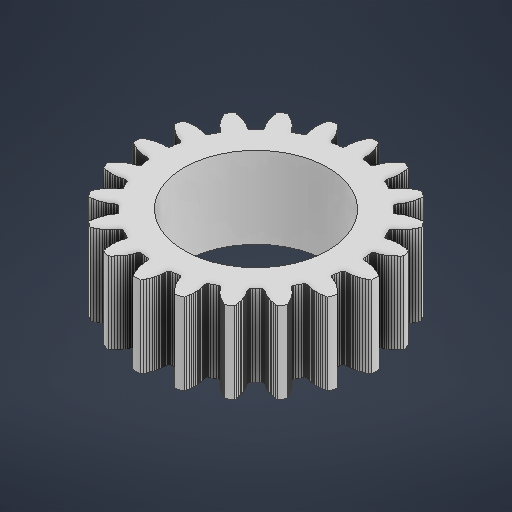
# Autodesk Inventor part: pole_gear_v2
Saved by Autodesk Inventor 2026.2 (Build 302298000, 298)
## iProperties
Created: 2026-01-14
Part Number: pole_gear_v2
Material: Generic
Document SubType Name: Modeling
Designer: User
Density: 1 g/cm^3
Appearance: Default
Author: User
Autodesk Inventor part; units mm, degrees
(part 1 of 3)
ref_plane "YZ Plane" through (0, 0, 0) normal (1, 0, 0) x (0, 1, 0)
ref_plane "XZ Plane" through (0, 0, 0) normal (0, 1, 0) x (-1, 0, 0)
ref_plane "XY Plane" through (0, 0, 0) normal (0, 0, 1) x (1, 0, 0)
sketch "Sketch1" plane through (0, 0, 0) normal (0, 1, 0) x (-1, 0, 0)
  circle A0 centre (0, 0) radius 13.25
  circle A1 centre (0, 0) radius 13.25
  line L0 (20.839, 5.8308) -> (20.5291, 5.5298)
  line L1 (20.5291, 5.5298) -> (20.2304, 5.263)
  line L2 (20.2304, 5.263) -> (19.9477, 5.0311)
  line L3 (19.9477, 5.0311) -> (19.6809, 4.8302)
  line L4 (19.6809, 4.8302) -> (19.4329, 4.6593)
  line L5 (19.4329, 4.6593) -> (19.2065, 4.5169)
  line L6 (19.2065, 4.5169) -> (19.0014, 4.3995)
  line L7 (19.0014, 4.3995) -> (18.8229, 4.307)
  line L8 (18.8229, 4.307) -> (18.5448, 4.1835)
  line L9 (18.5448, 4.1835) -> (18.3792, 4.1257)
  line L10 (18.3792, 4.1257) -> (18.2149, 4.0764)
  line L11 (18.2149, 4.0764) -> (18.015, 3.9979)
  line L12 (18.015, 3.9979) -> (17.8537, 3.9113)
  line L13 (17.8537, 3.9113) -> (17.7876, 3.866)
  line L14 (17.7876, 3.866) -> (17.7313, 3.8197)
  line L15 (17.7313, 3.8197) -> (17.6846, 3.773)
  line L16 (17.6846, 3.773) -> (17.6477, 3.7262)
  line L17 (17.6477, 3.7262) -> (17.6205, 3.6797)
  line L18 (17.6205, 3.6797) -> (17.6029, 3.6338)
  line L19 (17.6029, 3.6338) -> (17.5949, 3.589)
  line L20 (17.5949, 3.589) -> (17.5985, 3.5351)
  line L21 (17.5985, 3.5351) -> (17.6581, 3.2242)
  line L22 (17.6581, 3.2242) -> (17.729, 2.808)
  line L23 (17.729, 2.808) -> (17.7902, 2.3902)
  line L24 (17.7902, 2.3902) -> (17.8295, 2.0761)
  line L25 (17.8295, 2.0761) -> (17.8429, 2.0238)
  line L26 (17.8429, 2.0238) -> (17.8643, 1.9836)
  line L27 (17.8643, 1.9836) -> (17.8951, 1.9454)
  line L28 (17.8951, 1.9454) -> (17.9354, 1.9096)
  line L29 (17.9354, 1.9096) -> (17.985, 1.8765)
  line L30 (17.985, 1.8765) -> (18.0438, 1.8465)
  line L31 (18.0438, 1.8465) -> (18.1117, 1.8199)
  line L32 (18.1117, 1.8199) -> (18.1886, 1.7972)
  line L33 (18.1886, 1.7972) -> (18.3687, 1.7647)
  line L34 (18.3687, 1.7647) -> (18.583, 1.7518)
  line L35 (18.583, 1.7518) -> (18.7546, 1.7557)
  line L36 (18.7546, 1.7557) -> (18.9299, 1.7519)
  line L37 (18.9299, 1.7519) -> (19.2325, 1.7204)
  line L38 (19.2325, 1.7204) -> (19.4309, 1.6876)
  line L39 (19.4309, 1.6876) -> (19.6623, 1.6393)
  line L40 (19.6623, 1.6393) -> (19.9216, 1.5738)
  line L41 (19.9216, 1.5738) -> (20.2103, 1.4879)
  line L42 (20.2103, 1.4879) -> (20.5261, 1.3793)
  line L43 (20.5261, 1.3793) -> (20.8666, 1.2461)
  line L44 (20.8666, 1.2461) -> (21.2331, 1.0847)
  line L45 (21.2331, 1.0847) -> (21.6209, 0.8942)
  line L46 (21.6209, 0.8942) -> (21.989, 0.6945)
  arc A2 (21.989, -0.6945) -> (21.989, 0.6945) centre (0, 0) ccw
  line L47 (21.989, -0.6945) -> (21.6209, -0.8942)
  line L48 (21.6209, -0.8942) -> (21.2331, -1.0847)
  line L49 (21.2331, -1.0847) -> (20.8666, -1.2461)
  line L50 (20.8666, -1.2461) -> (20.5261, -1.3793)
  line L51 (20.5261, -1.3793) -> (20.2103, -1.4879)
  line L52 (20.2103, -1.4879) -> (19.9216, -1.5738)
  line L53 (19.9216, -1.5738) -> (19.6623, -1.6393)
  line L54 (19.6623, -1.6393) -> (19.4309, -1.6876)
  line L55 (19.4309, -1.6876) -> (19.2325, -1.7204)
  line L56 (19.2325, -1.7204) -> (18.9299, -1.7519)
  line L57 (18.9299, -1.7519) -> (18.7546, -1.7557)
  line L58 (18.7546, -1.7557) -> (18.583, -1.7518)
  line L59 (18.583, -1.7518) -> (18.3687, -1.7647)
  line L60 (18.3687, -1.7647) -> (18.1886, -1.7972)
  line L61 (18.1886, -1.7972) -> (18.1117, -1.8199)
  line L62 (18.1117, -1.8199) -> (18.0438, -1.8465)
  line L63 (18.0438, -1.8465) -> (17.985, -1.8765)
  line L64 (17.985, -1.8765) -> (17.9354, -1.9096)
  line L65 (17.9354, -1.9096) -> (17.8951, -1.9454)
  line L66 (17.8951, -1.9454) -> (17.8643, -1.9836)
  line L67 (17.8643, -1.9836) -> (17.8429, -2.0238)
  line L68 (17.8429, -2.0238) -> (17.8295, -2.0761)
  line L69 (17.8295, -2.0761) -> (17.7902, -2.3902)
  line L70 (17.7902, -2.3902) -> (17.729, -2.808)
  line L71 (17.729, -2.808) -> (17.6581, -3.2242)
  line L72 (17.6581, -3.2242) -> (17.5985, -3.5351)
  line L73 (17.5985, -3.5351) -> (17.5949, -3.589)
  line L74 (17.5949, -3.589) -> (17.6029, -3.6338)
  line L75 (17.6029, -3.6338) -> (17.6205, -3.6797)
  line L76 (17.6205, -3.6797) -> (17.6477, -3.7262)
  line L77 (17.6477, -3.7262) -> (17.6846, -3.773)
  line L78 (17.6846, -3.773) -> (17.7313, -3.8197)
  line L79 (17.7313, -3.8197) -> (17.7876, -3.866)
  line L80 (17.7876, -3.866) -> (17.8537, -3.9113)
  line L81 (17.8537, -3.9113) -> (18.015, -3.9979)
  line L82 (18.015, -3.9979) -> (18.2149, -4.0764)
  line L83 (18.2149, -4.0764) -> (18.3792, -4.1257)
  line L84 (18.3792, -4.1257) -> (18.5448, -4.1835)
  line L85 (18.5448, -4.1835) -> (18.8229, -4.307)
  line L86 (18.8229, -4.307) -> (19.0014, -4.3995)
  line L87 (19.0014, -4.3995) -> (19.2065, -4.5169)
  line L88 (19.2065, -4.5169) -> (19.4329, -4.6593)
  line L89 (19.4329, -4.6593) -> (19.6809, -4.8302)
  line L90 (19.6809, -4.8302) -> (19.9477, -5.0311)
  line L91 (19.9477, -5.0311) -> (20.2304, -5.263)
  line L92 (20.2304, -5.263) -> (20.5291, -5.5298)
  line L93 (20.5291, -5.5298) -> (20.839, -5.8308)
  line L94 (20.839, -5.8308) -> (21.1274, -6.1345)
  arc A3 (20.6982, -7.4555) -> (21.1274, -6.1345) centre (0, 0) ccw
  line L95 (20.6982, -7.4555) -> (20.2864, -7.5317)
  line L96 (20.2864, -7.5317) -> (19.8587, -7.593)
  line L97 (19.8587, -7.593) -> (19.4602, -7.6332)
  line L98 (19.4602, -7.6332) -> (19.0953, -7.6547)
  line L99 (19.0953, -7.6547) -> (18.7613, -7.6604)
  line L100 (18.7613, -7.6604) -> (18.4602, -7.6529)
  line L101 (18.4602, -7.6529) -> (18.1934, -7.6351)
  line L102 (18.1934, -7.6351) -> (17.9584, -7.6095)
  line L103 (17.9584, -7.6095) -> (17.7596, -7.5794)
  line L104 (17.7596, -7.5794) -> (17.462, -7.5158)
  line L105 (17.462, -7.5158) -> (17.2942, -7.4653)
  line L106 (17.2942, -7.4653) -> (17.1322, -7.4085)
  line L107 (17.1322, -7.4085) -> (16.9244, -7.3546)
  line L108 (16.9244, -7.3546) -> (16.743, -7.3298)
  line L109 (16.743, -7.3298) -> (16.6629, -7.3277)
  line L110 (16.6629, -7.3277) -> (16.5901, -7.3319)
  line L111 (16.5901, -7.3319) -> (16.5249, -7.3423)
  line L112 (16.5249, -7.3423) -> (16.4675, -7.3585)
  line L113 (16.4675, -7.3585) -> (16.4181, -7.3801)
  line L114 (16.4181, -7.3801) -> (16.3769, -7.4069)
  line L115 (16.3769, -7.4069) -> (16.3442, -7.4385)
  line L116 (16.3442, -7.4385) -> (16.3153, -7.4841)
  line L117 (16.3153, -7.4841) -> (16.1809, -7.7707)
  line L118 (16.1809, -7.7707) -> (15.9936, -8.1491)
  line L119 (15.9936, -8.1491) -> (15.7975, -8.5231)
  line L120 (15.7975, -8.5231) -> (15.6447, -8.8003)
  line L121 (15.6447, -8.8003) -> (15.6247, -8.8505)
  line L122 (15.6247, -8.8505) -> (15.6184, -8.8956)
  line L123 (15.6184, -8.8956) -> (15.621, -8.9446)
  line L124 (15.621, -8.9446) -> (15.6325, -8.9973)
  line L125 (15.6325, -8.9973) -> (15.6531, -9.0532)
  line L126 (15.6531, -9.0532) -> (15.6831, -9.112)
  line L127 (15.6831, -9.112) -> (15.7224, -9.1734)
  line L128 (15.7224, -9.1734) -> (15.7712, -9.237)
  line L129 (15.7712, -9.237) -> (15.8979, -9.3692)
  line L130 (15.8979, -9.3692) -> (16.0637, -9.5056)
  line L131 (16.0637, -9.5056) -> (16.2048, -9.6033)
  line L132 (16.2048, -9.6033) -> (16.3443, -9.7094)
  line L133 (16.3443, -9.7094) -> (16.5707, -9.9128)
  line L134 (16.5707, -9.9128) -> (16.7119, -10.0559)
  line L135 (16.7119, -10.0559) -> (16.8707, -10.231)
  line L136 (16.8707, -10.231) -> (17.042, -10.4364)
  line L137 (17.042, -10.4364) -> (17.225, -10.6756)
  line L138 (17.225, -10.6756) -> (17.4167, -10.9491)
  line L139 (17.4167, -10.9491) -> (17.6139, -11.257)
  line L140 (17.6139, -11.257) -> (17.8155, -11.603)
  line L141 (17.8155, -11.603) -> (18.0173, -11.985)
  line L142 (18.0173, -11.985) -> (18.1977, -12.3629)
  arc A4 (17.3813, -13.4867) -> (18.1977, -12.3629) centre (0, 0) ccw
  line L143 (17.3813, -13.4867) -> (16.9661, -13.4319)
  line L144 (16.9661, -13.4319) -> (16.5404, -13.3581)
  line L145 (16.5404, -13.3581) -> (16.149, -13.2732)
  line L146 (16.149, -13.2732) -> (15.7953, -13.1808)
  line L147 (15.7953, -13.1808) -> (15.4759, -13.083)
  line L148 (15.4759, -13.083) -> (15.1918, -12.9829)
  line L149 (15.1918, -12.9829) -> (14.9436, -12.8835)
  line L150 (14.9436, -12.8835) -> (14.728, -12.7865)
  line L151 (14.728, -12.7865) -> (14.5482, -12.6964)
  line L152 (14.5482, -12.6964) -> (14.2849, -12.544)
  line L153 (14.2849, -12.544) -> (14.1408, -12.4441)
  line L154 (14.1408, -12.4441) -> (14.0043, -12.3401)
  line L155 (14.0043, -12.3401) -> (13.8234, -12.2245)
  line L156 (13.8234, -12.2245) -> (13.6585, -12.1449)
  line L157 (13.6585, -12.1449) -> (13.5829, -12.1181)
  line L158 (13.5829, -12.1181) -> (13.5124, -12.0997)
  line L159 (13.5124, -12.0997) -> (13.4472, -12.0894)
  line L160 (13.4472, -12.0894) -> (13.3876, -12.0871)
  line L161 (13.3876, -12.0871) -> (13.334, -12.0924)
  line L162 (13.334, -12.0924) -> (13.2865, -12.1051)
  line L163 (13.2865, -12.1051) -> (13.2456, -12.125)
  line L164 (13.2456, -12.125) -> (13.2041, -12.1596)
  line L165 (13.2041, -12.1596) -> (12.9876, -12.3906)
  line L166 (12.9876, -12.3906) -> (12.6926, -12.6926)
  line L167 (12.6926, -12.6926) -> (12.3906, -12.9876)
  line L168 (12.3906, -12.9876) -> (12.1596, -13.2041)
  line L169 (12.1596, -13.2041) -> (12.125, -13.2456)
  line L170 (12.125, -13.2456) -> (12.1051, -13.2865)
  line L171 (12.1051, -13.2865) -> (12.0924, -13.334)
  line L172 (12.0924, -13.334) -> (12.0871, -13.3876)
  line L173 (12.0871, -13.3876) -> (12.0894, -13.4472)
  line L174 (12.0894, -13.4472) -> (12.0997, -13.5124)
  line L175 (12.0997, -13.5124) -> (12.1181, -13.5829)
  line L176 (12.1181, -13.5829) -> (12.1449, -13.6585)
  line L177 (12.1449, -13.6585) -> (12.2245, -13.8234)
  line L178 (12.2245, -13.8234) -> (12.3401, -14.0043)
  line L179 (12.3401, -14.0043) -> (12.4441, -14.1408)
  line L180 (12.4441, -14.1408) -> (12.544, -14.2849)
  line L181 (12.544, -14.2849) -> (12.6964, -14.5482)
  line L182 (12.6964, -14.5482) -> (12.7865, -14.728)
  line L183 (12.7865, -14.728) -> (12.8835, -14.9436)
  line L184 (12.8835, -14.9436) -> (12.9829, -15.1918)
  line L185 (12.9829, -15.1918) -> (13.083, -15.4759)
  line L186 (13.083, -15.4759) -> (13.1808, -15.7953)
  line L187 (13.1808, -15.7953) -> (13.2732, -16.149)
  line L188 (13.2732, -16.149) -> (13.3581, -16.5404)
  line L189 (13.3581, -16.5404) -> (13.4319, -16.9661)
  line L190 (13.4319, -16.9661) -> (13.4867, -17.3813)
  arc A5 (12.3629, -18.1977) -> (13.4867, -17.3813) centre (0, 0) ccw
  line L191 (12.3629, -18.1977) -> (11.985, -18.0173)
  line L192 (11.985, -18.0173) -> (11.603, -17.8155)
  line L193 (11.603, -17.8155) -> (11.257, -17.6139)
  line L194 (11.257, -17.6139) -> (10.9491, -17.4167)
  line L195 (10.9491, -17.4167) -> (10.6756, -17.225)
  line L196 (10.6756, -17.225) -> (10.4364, -17.042)
  line L197 (10.4364, -17.042) -> (10.231, -16.8707)
  line L198 (10.231, -16.8707) -> (10.0559, -16.7119)
  line L199 (10.0559, -16.7119) -> (9.9128, -16.5707)
  line L200 (9.9128, -16.5707) -> (9.7094, -16.3443)
  line L201 (9.7094, -16.3443) -> (9.6033, -16.2048)
  line L202 (9.6033, -16.2048) -> (9.5056, -16.0637)
  line L203 (9.5056, -16.0637) -> (9.3692, -15.8979)
  line L204 (9.3692, -15.8979) -> (9.237, -15.7712)
  line L205 (9.237, -15.7712) -> (9.1734, -15.7224)
  line L206 (9.1734, -15.7224) -> (9.112, -15.6831)
  line L207 (9.112, -15.6831) -> (9.0532, -15.6531)
  line L208 (9.0532, -15.6531) -> (8.9973, -15.6325)
  line L209 (8.9973, -15.6325) -> (8.9446, -15.621)
  line L210 (8.9446, -15.621) -> (8.8956, -15.6184)
  line L211 (8.8956, -15.6184) -> (8.8505, -15.6247)
  line L212 (8.8505, -15.6247) -> (8.8003, -15.6447)
  line L213 (8.8003, -15.6447) -> (8.5231, -15.7975)
  line L214 (8.5231, -15.7975) -> (8.1491, -15.9936)
  line L215 (8.1491, -15.9936) -> (7.7707, -16.1809)
  line L216 (7.7707, -16.1809) -> (7.4841, -16.3153)
  line L217 (7.4841, -16.3153) -> (7.4385, -16.3442)
  line L218 (7.4385, -16.3442) -> (7.4069, -16.3769)
  line L219 (7.4069, -16.3769) -> (7.3801, -16.4181)
  line L220 (7.3801, -16.4181) -> (7.3585, -16.4675)
  line L221 (7.3585, -16.4675) -> (7.3423, -16.5249)
  line L222 (7.3423, -16.5249) -> (7.3319, -16.5901)
  line L223 (7.3319, -16.5901) -> (7.3277, -16.6629)
  line L224 (7.3277, -16.6629) -> (7.3298, -16.743)
  line L225 (7.3298, -16.743) -> (7.3546, -16.9244)
  line L226 (7.3546, -16.9244) -> (7.4085, -17.1322)
  line L227 (7.4085, -17.1322) -> (7.4653, -17.2942)
  line L228 (7.4653, -17.2942) -> (7.5158, -17.462)
  line L229 (7.5158, -17.462) -> (7.5794, -17.7596)
  line L230 (7.5794, -17.7596) -> (7.6095, -17.9584)
  line L231 (7.6095, -17.9584) -> (7.6351, -18.1934)
  line L232 (7.6351, -18.1934) -> (7.6529, -18.4602)
  line L233 (7.6529, -18.4602) -> (7.6604, -18.7613)
  line L234 (7.6604, -18.7613) -> (7.6547, -19.0953)
  line L235 (7.6547, -19.0953) -> (7.6332, -19.4602)
  line L236 (7.6332, -19.4602) -> (7.593, -19.8587)
  line L237 (7.593, -19.8587) -> (7.5317, -20.2864)
  line L238 (7.5317, -20.2864) -> (7.4555, -20.6982)
  arc A6 (6.1345, -21.1274) -> (7.4555, -20.6982) centre (0, 0) ccw
  line L239 (6.1345, -21.1274) -> (5.8308, -20.839)
  line L240 (5.8308, -20.839) -> (5.5298, -20.5291)
  line L241 (5.5298, -20.5291) -> (5.263, -20.2304)
  line L242 (5.263, -20.2304) -> (5.0311, -19.9477)
  line L243 (5.0311, -19.9477) -> (4.8302, -19.6809)
  line L244 (4.8302, -19.6809) -> (4.6593, -19.4329)
  line L245 (4.6593, -19.4329) -> (4.5169, -19.2065)
  line L246 (4.5169, -19.2065) -> (4.3995, -19.0014)
  line L247 (4.3995, -19.0014) -> (4.307, -18.8229)
  line L248 (4.307, -18.8229) -> (4.1835, -18.5448)
  line L249 (4.1835, -18.5448) -> (4.1257, -18.3792)
  line L250 (4.1257, -18.3792) -> (4.0764, -18.2149)
  line L251 (4.0764, -18.2149) -> (3.9979, -18.015)
  line L252 (3.9979, -18.015) -> (3.9113, -17.8537)
  line L253 (3.9113, -17.8537) -> (3.866, -17.7876)
  line L254 (3.866, -17.7876) -> (3.8197, -17.7313)
  line L255 (3.8197, -17.7313) -> (3.773, -17.6846)
  line L256 (3.773, -17.6846) -> (3.7262, -17.6477)
  line L257 (3.7262, -17.6477) -> (3.6797, -17.6205)
  line L258 (3.6797, -17.6205) -> (3.6338, -17.6029)
  line L259 (3.6338, -17.6029) -> (3.589, -17.5949)
  line L260 (3.589, -17.5949) -> (3.5351, -17.5985)
  line L261 (3.5351, -17.5985) -> (3.2242, -17.6581)
  line L262 (3.2242, -17.6581) -> (2.808, -17.729)
  line L263 (2.808, -17.729) -> (2.3902, -17.7902)
  line L264 (2.3902, -17.7902) -> (2.0761, -17.8295)
  line L265 (2.0761, -17.8295) -> (2.0238, -17.8429)
  line L266 (2.0238, -17.8429) -> (1.9836, -17.8643)
  line L267 (1.9836, -17.8643) -> (1.9454, -17.8951)
  line L268 (1.9454, -17.8951) -> (1.9096, -17.9354)
  line L269 (1.9096, -17.9354) -> (1.8765, -17.985)
  line L270 (1.8765, -17.985) -> (1.8465, -18.0438)
  line L271 (1.8465, -18.0438) -> (1.8199, -18.1117)
  line L272 (1.8199, -18.1117) -> (1.7972, -18.1886)
  line L273 (1.7972, -18.1886) -> (1.7647, -18.3687)
  line L274 (1.7647, -18.3687) -> (1.7518, -18.583)
  line L275 (1.7518, -18.583) -> (1.7557, -18.7546)
  line L276 (1.7557, -18.7546) -> (1.7519, -18.9299)
  line L277 (1.7519, -18.9299) -> (1.7204, -19.2325)
  line L278 (1.7204, -19.2325) -> (1.6876, -19.4309)
  line L279 (1.6876, -19.4309) -> (1.6393, -19.6623)
  line L280 (1.6393, -19.6623) -> (1.5738, -19.9216)
  line L281 (1.5738, -19.9216) -> (1.4879, -20.2103)
  line L282 (1.4879, -20.2103) -> (1.3793, -20.5261)
  line L283 (1.3793, -20.5261) -> (1.2461, -20.8666)
  line L284 (1.2461, -20.8666) -> (1.0847, -21.2331)
  line L285 (1.0847, -21.2331) -> (0.8942, -21.6209)
  line L286 (0.8942, -21.6209) -> (0.6945, -21.989)
  arc A7 (-0.6945, -21.989) -> (0.6945, -21.989) centre (0, 0) ccw
  line L287 (-0.6945, -21.989) -> (-0.8942, -21.6209)
  line L288 (-0.8942, -21.6209) -> (-1.0847, -21.2331)
  line L289 (-1.0847, -21.2331) -> (-1.2461, -20.8666)
  line L290 (-1.2461, -20.8666) -> (-1.3793, -20.5261)
  line L291 (-1.3793, -20.5261) -> (-1.4879, -20.2103)
  line L292 (-1.4879, -20.2103) -> (-1.5738, -19.9216)
  line L293 (-1.5738, -19.9216) -> (-1.6393, -19.6623)
  line L294 (-1.6393, -19.6623) -> (-1.6876, -19.4309)
  line L295 (-1.6876, -19.4309) -> (-1.7204, -19.2325)
  line L296 (-1.7204, -19.2325) -> (-1.7519, -18.9299)
  line L297 (-1.7519, -18.9299) -> (-1.7557, -18.7546)
  line L298 (-1.7557, -18.7546) -> (-1.7518, -18.583)
  line L299 (-1.7518, -18.583) -> (-1.7647, -18.3687)
  line L300 (-1.7647, -18.3687) -> (-1.7972, -18.1886)
  line L301 (-1.7972, -18.1886) -> (-1.8199, -18.1117)
  line L302 (-1.8199, -18.1117) -> (-1.8465, -18.0438)
  line L303 (-1.8465, -18.0438) -> (-1.8765, -17.985)
  line L304 (-1.8765, -17.985) -> (-1.9096, -17.9354)
  line L305 (-1.9096, -17.9354) -> (-1.9454, -17.8951)
  line L306 (-1.9454, -17.8951) -> (-1.9836, -17.8643)
  line L307 (-1.9836, -17.8643) -> (-2.0238, -17.8429)
  line L308 (-2.0238, -17.8429) -> (-2.0761, -17.8295)
  line L309 (-2.0761, -17.8295) -> (-2.3902, -17.7902)
  line L310 (-2.3902, -17.7902) -> (-2.808, -17.729)
  line L311 (-2.808, -17.729) -> (-3.2242, -17.6581)
  line L312 (-3.2242, -17.6581) -> (-3.5351, -17.5985)
  line L313 (-3.5351, -17.5985) -> (-3.589, -17.5949)
  line L314 (-3.589, -17.5949) -> (-3.6338, -17.6029)
  line L315 (-3.6338, -17.6029) -> (-3.6797, -17.6205)
  line L316 (-3.6797, -17.6205) -> (-3.7262, -17.6477)
  line L317 (-3.7262, -17.6477) -> (-3.773, -17.6846)
  line L318 (-3.773, -17.6846) -> (-3.8197, -17.7313)
  line L319 (-3.8197, -17.7313) -> (-3.866, -17.7876)
  line L320 (-3.866, -17.7876) -> (-3.9113, -17.8537)
  line L321 (-3.9113, -17.8537) -> (-3.9979, -18.015)
  line L322 (-3.9979, -18.015) -> (-4.0764, -18.2149)
  line L323 (-4.0764, -18.2149) -> (-4.1257, -18.3792)
  line L324 (-4.1257, -18.3792) -> (-4.1835, -18.5448)
  line L325 (-4.1835, -18.5448) -> (-4.307, -18.8229)
  line L326 (-4.307, -18.8229) -> (-4.3995, -19.0014)
  line L327 (-4.3995, -19.0014) -> (-4.5169, -19.2065)
  line L328 (-4.5169, -19.2065) -> (-4.6593, -19.4329)
  line L329 (-4.6593, -19.4329) -> (-4.8302, -19.6809)
  line L330 (-4.8302, -19.6809) -> (-5.0311, -19.9477)
  line L331 (-5.0311, -19.9477) -> (-5.263, -20.2304)
  line L332 (-5.263, -20.2304) -> (-5.5298, -20.5291)
  line L333 (-5.5298, -20.5291) -> (-5.8308, -20.839)
  line L334 (-5.8308, -20.839) -> (-6.1345, -21.1274)
  arc A8 (-7.4555, -20.6982) -> (-6.1345, -21.1274) centre (0, 0) ccw
  line L335 (-7.4555, -20.6982) -> (-7.5317, -20.2864)
  line L336 (-7.5317, -20.2864) -> (-7.593, -19.8587)
  line L337 (-7.593, -19.8587) -> (-7.6332, -19.4602)
  line L338 (-7.6332, -19.4602) -> (-7.6547, -19.0953)
  line L339 (-7.6547, -19.0953) -> (-7.6604, -18.7613)
  line L340 (-7.6604, -18.7613) -> (-7.6529, -18.4602)
  line L341 (-7.6529, -18.4602) -> (-7.6351, -18.1934)
  line L342 (-7.6351, -18.1934) -> (-7.6095, -17.9584)
  line L343 (-7.6095, -17.9584) -> (-7.5794, -17.7596)
  line L344 (-7.5794, -17.7596) -> (-7.5158, -17.462)
  line L345 (-7.5158, -17.462) -> (-7.4653, -17.2942)
  line L346 (-7.4653, -17.2942) -> (-7.4085, -17.1322)
  line L347 (-7.4085, -17.1322) -> (-7.3546, -16.9244)
  line L348 (-7.3546, -16.9244) -> (-7.3298, -16.743)
  line L349 (-7.3298, -16.743) -> (-7.3277, -16.6629)
  line L350 (-7.3277, -16.6629) -> (-7.3319, -16.5901)
  line L351 (-7.3319, -16.5901) -> (-7.3423, -16.5249)
  line L352 (-7.3423, -16.5249) -> (-7.3585, -16.4675)
  line L353 (-7.3585, -16.4675) -> (-7.3801, -16.4181)
  line L354 (-7.3801, -16.4181) -> (-7.4069, -16.3769)
  line L355 (-7.4069, -16.3769) -> (-7.4385, -16.3442)
  line L356 (-7.4385, -16.3442) -> (-7.4841, -16.3153)
  line L357 (-7.4841, -16.3153) -> (-7.7707, -16.1809)
  line L358 (-7.7707, -16.1809) -> (-8.1491, -15.9936)
  line L359 (-8.1491, -15.9936) -> (-8.5231, -15.7975)
  line L360 (-8.5231, -15.7975) -> (-8.8003, -15.6447)
  line L361 (-8.8003, -15.6447) -> (-8.8505, -15.6247)
  line L362 (-8.8505, -15.6247) -> (-8.8956, -15.6184)
  line L363 (-8.8956, -15.6184) -> (-8.9446, -15.621)
  line L364 (-8.9446, -15.621) -> (-8.9973, -15.6325)
  line L365 (-8.9973, -15.6325) -> (-9.0532, -15.6531)
  line L366 (-9.0532, -15.6531) -> (-9.112, -15.6831)
  line L367 (-9.112, -15.6831) -> (-9.1734, -15.7224)
  line L368 (-9.1734, -15.7224) -> (-9.237, -15.7712)
  line L369 (-9.237, -15.7712) -> (-9.3692, -15.8979)
  line L370 (-9.3692, -15.8979) -> (-9.5056, -16.0637)
  line L371 (-9.5056, -16.0637) -> (-9.6033, -16.2048)
  line L372 (-9.6033, -16.2048) -> (-9.7094, -16.3443)
  line L373 (-9.7094, -16.3443) -> (-9.9128, -16.5707)
  line L374 (-9.9128, -16.5707) -> (-10.0559, -16.7119)
  line L375 (-10.0559, -16.7119) -> (-10.231, -16.8707)
  line L376 (-10.231, -16.8707) -> (-10.4364, -17.042)
  line L377 (-10.4364, -17.042) -> (-10.6756, -17.225)
  line L378 (-10.6756, -17.225) -> (-10.9491, -17.4167)
  line L379 (-10.9491, -17.4167) -> (-11.257, -17.6139)
  line L380 (-11.257, -17.6139) -> (-11.603, -17.8155)
  line L381 (-11.603, -17.8155) -> (-11.985, -18.0173)
  line L382 (-11.985, -18.0173) -> (-12.3629, -18.1977)
  arc A9 (-13.4867, -17.3813) -> (-12.3629, -18.1977) centre (0, 0) ccw
  line L383 (-13.4867, -17.3813) -> (-13.4319, -16.9661)
  line L384 (-13.4319, -16.9661) -> (-13.3581, -16.5404)
  line L385 (-13.3581, -16.5404) -> (-13.2732, -16.149)
  line L386 (-13.2732, -16.149) -> (-13.1808, -15.7953)
  line L387 (-13.1808, -15.7953) -> (-13.083, -15.4759)
  line L388 (-13.083, -15.4759) -> (-12.9829, -15.1918)
  line L389 (-12.9829, -15.1918) -> (-12.8835, -14.9436)
  line L390 (-12.8835, -14.9436) -> (-12.7865, -14.728)
  line L391 (-12.7865, -14.728) -> (-12.6964, -14.5482)
  line L392 (-12.6964, -14.5482) -> (-12.544, -14.2849)
  line L393 (-12.544, -14.2849) -> (-12.4441, -14.1408)
  line L394 (-12.4441, -14.1408) -> (-12.3401, -14.0043)
  line L395 (-12.3401, -14.0043) -> (-12.2245, -13.8234)
  line L396 (-12.2245, -13.8234) -> (-12.1449, -13.6585)
  line L397 (-12.1449, -13.6585) -> (-12.1181, -13.5829)
  line L398 (-12.1181, -13.5829) -> (-12.0997, -13.5124)
  line L399 (-12.0997, -13.5124) -> (-12.0894, -13.4472)
  line L400 (-12.0894, -13.4472) -> (-12.0871, -13.3876)
  line L401 (-12.0871, -13.3876) -> (-12.0924, -13.334)
  line L402 (-12.0924, -13.334) -> (-12.1051, -13.2865)
  line L403 (-12.1051, -13.2865) -> (-12.125, -13.2456)
  line L404 (-12.125, -13.2456) -> (-12.1596, -13.2041)
  line L405 (-12.1596, -13.2041) -> (-12.3906, -12.9876)
  line L406 (-12.3906, -12.9876) -> (-12.6926, -12.6926)
  line L407 (-12.6926, -12.6926) -> (-12.9876, -12.3906)
  line L408 (-12.9876, -12.3906) -> (-13.2041, -12.1596)
  line L409 (-13.2041, -12.1596) -> (-13.2456, -12.125)
  line L410 (-13.2456, -12.125) -> (-13.2865, -12.1051)
  line L411 (-13.2865, -12.1051) -> (-13.334, -12.0924)
  line L412 (-13.334, -12.0924) -> (-13.3876, -12.0871)
  line L413 (-13.3876, -12.0871) -> (-13.4472, -12.0894)
  line L414 (-13.4472, -12.0894) -> (-13.5124, -12.0997)
  line L415 (-13.5124, -12.0997) -> (-13.5829, -12.1181)
  line L416 (-13.5829, -12.1181) -> (-13.6585, -12.1449)
  line L417 (-13.6585, -12.1449) -> (-13.8234, -12.2245)
  line L418 (-13.8234, -12.2245) -> (-14.0043, -12.3401)
  line L419 (-14.0043, -12.3401) -> (-14.1408, -12.4441)
  line L420 (-14.1408, -12.4441) -> (-14.2849, -12.544)
  line L421 (-14.2849, -12.544) -> (-14.5482, -12.6964)
  line L422 (-14.5482, -12.6964) -> (-14.728, -12.7865)
  line L423 (-14.728, -12.7865) -> (-14.9436, -12.8835)
  line L424 (-14.9436, -12.8835) -> (-15.1918, -12.9829)
  line L425 (-15.1918, -12.9829) -> (-15.4759, -13.083)
  line L426 (-15.4759, -13.083) -> (-15.7953, -13.1808)
  line L427 (-15.7953, -13.1808) -> (-16.149, -13.2732)
  line L428 (-16.149, -13.2732) -> (-16.5404, -13.3581)
  line L429 (-16.5404, -13.3581) -> (-16.9661, -13.4319)
  line L430 (-16.9661, -13.4319) -> (-17.3813, -13.4867)
  arc A10 (-18.1977, -12.3629) -> (-17.3813, -13.4867) centre (0, 0) ccw
  line L431 (-18.1977, -12.3629) -> (-18.0173, -11.985)
  line L432 (-18.0173, -11.985) -> (-17.8155, -11.603)
  line L433 (-17.8155, -11.603) -> (-17.6139, -11.257)
  line L434 (-17.6139, -11.257) -> (-17.4167, -10.9491)
  line L435 (-17.4167, -10.9491) -> (-17.225, -10.6756)
  line L436 (-17.225, -10.6756) -> (-17.042, -10.4364)
  line L437 (-17.042, -10.4364) -> (-16.8707, -10.231)
  line L438 (-16.8707, -10.231) -> (-16.7119, -10.0559)
  line L439 (-16.7119, -10.0559) -> (-16.5707, -9.9128)
  line L440 (-16.5707, -9.9128) -> (-16.3443, -9.7094)
  line L441 (-16.3443, -9.7094) -> (-16.2048, -9.6033)
  line L442 (-16.2048, -9.6033) -> (-16.0637, -9.5056)
  line L443 (-16.0637, -9.5056) -> (-15.8979, -9.3692)
  line L444 (-15.8979, -9.3692) -> (-15.7712, -9.237)
  line L445 (-15.7712, -9.237) -> (-15.7224, -9.1734)
  line L446 (-15.7224, -9.1734) -> (-15.6831, -9.112)
  line L447 (-15.6831, -9.112) -> (-15.6531, -9.0532)
  line L448 (-15.6531, -9.0532) -> (-15.6325, -8.9973)
  line L449 (-15.6325, -8.9973) -> (-15.621, -8.9446)
  line L450 (-15.621, -8.9446) -> (-15.6184, -8.8956)
  line L451 (-15.6184, -8.8956) -> (-15.6247, -8.8505)
  line L452 (-15.6247, -8.8505) -> (-15.6447, -8.8003)
  line L453 (-15.6447, -8.8003) -> (-15.7975, -8.5231)
  line L454 (-15.7975, -8.5231) -> (-15.9936, -8.1491)
  line L455 (-15.9936, -8.1491) -> (-16.1809, -7.7707)
  line L456 (-16.1809, -7.7707) -> (-16.3153, -7.4841)
  line L457 (-16.3153, -7.4841) -> (-16.3442, -7.4385)
  line L458 (-16.3442, -7.4385) -> (-16.3769, -7.4069)
  line L459 (-16.3769, -7.4069) -> (-16.4181, -7.3801)
  line L460 (-16.4181, -7.3801) -> (-16.4675, -7.3585)
  line L461 (-16.4675, -7.3585) -> (-16.5249, -7.3423)
  line L462 (-16.5249, -7.3423) -> (-16.5901, -7.3319)
  line L463 (-16.5901, -7.3319) -> (-16.6629, -7.3277)
  line L464 (-16.6629, -7.3277) -> (-16.743, -7.3298)
  line L465 (-16.743, -7.3298) -> (-16.9244, -7.3546)
  line L466 (-16.9244, -7.3546) -> (-17.1322, -7.4085)
  line L467 (-17.1322, -7.4085) -> (-17.2942, -7.4653)
  line L468 (-17.2942, -7.4653) -> (-17.462, -7.5158)
  line L469 (-17.462, -7.5158) -> (-17.7596, -7.5794)
  line L470 (-17.7596, -7.5794) -> (-17.9584, -7.6095)
  line L471 (-17.9584, -7.6095) -> (-18.1934, -7.6351)
  line L472 (-18.1934, -7.6351) -> (-18.4602, -7.6529)
  line L473 (-18.4602, -7.6529) -> (-18.7613, -7.6604)
  line L474 (-18.7613, -7.6604) -> (-19.0953, -7.6547)
  line L475 (-19.0953, -7.6547) -> (-19.4602, -7.6332)
  line L476 (-19.4602, -7.6332) -> (-19.8587, -7.593)
  line L477 (-19.8587, -7.593) -> (-20.2864, -7.5317)
  line L478 (-20.2864, -7.5317) -> (-20.6982, -7.4555)
  arc A11 (-21.1274, -6.1345) -> (-20.6982, -7.4555) centre (0, 0) ccw
  line L479 (-21.1274, -6.1345) -> (-20.839, -5.8308)
  line L480 (-20.839, -5.8308) -> (-20.5291, -5.5298)
  line L481 (-20.5291, -5.5298) -> (-20.2304, -5.263)
  line L482 (-20.2304, -5.263) -> (-19.9477, -5.0311)
  line L483 (-19.9477, -5.0311) -> (-19.6809, -4.8302)
  line L484 (-19.6809, -4.8302) -> (-19.4329, -4.6593)
  line L485 (-19.4329, -4.6593) -> (-19.2065, -4.5169)
  line L486 (-19.2065, -4.5169) -> (-19.0014, -4.3995)
  line L487 (-19.0014, -4.3995) -> (-18.8229, -4.307)
  line L488 (-18.8229, -4.307) -> (-18.5448, -4.1835)
  line L489 (-18.5448, -4.1835) -> (-18.3792, -4.1257)
  line L490 (-18.3792, -4.1257) -> (-18.2149, -4.0764)
  line L491 (-18.2149, -4.0764) -> (-18.015, -3.9979)
  line L492 (-18.015, -3.9979) -> (-17.8537, -3.9113)
  line L493 (-17.8537, -3.9113) -> (-17.7876, -3.866)
  line L494 (-17.7876, -3.866) -> (-17.7313, -3.8197)
  line L495 (-17.7313, -3.8197) -> (-17.6846, -3.773)
  line L496 (-17.6846, -3.773) -> (-17.6477, -3.7262)
  line L497 (-17.6477, -3.7262) -> (-17.6205, -3.6797)
  line L498 (-17.6205, -3.6797) -> (-17.6029, -3.6338)
  line L499 (-17.6029, -3.6338) -> (-17.5949, -3.589)
  line L500 (-17.5949, -3.589) -> (-17.5985, -3.5351)
  line L501 (-17.5985, -3.5351) -> (-17.6581, -3.2242)
  line L502 (-17.6581, -3.2242) -> (-17.729, -2.808)
  line L503 (-17.729, -2.808) -> (-17.7902, -2.3902)
  line L504 (-17.7902, -2.3902) -> (-17.8295, -2.0761)
  line L505 (-17.8295, -2.0761) -> (-17.8429, -2.0238)
  line L506 (-17.8429, -2.0238) -> (-17.8643, -1.9836)
  line L507 (-17.8643, -1.9836) -> (-17.8951, -1.9454)
  line L508 (-17.8951, -1.9454) -> (-17.9354, -1.9096)
  line L509 (-17.9354, -1.9096) -> (-17.985, -1.8765)
  line L510 (-17.985, -1.8765) -> (-18.0438, -1.8465)
  line L511 (-18.0438, -1.8465) -> (-18.1117, -1.8199)
  line L512 (-18.1117, -1.8199) -> (-18.1886, -1.7972)
  line L513 (-18.1886, -1.7972) -> (-18.3687, -1.7647)
  line L514 (-18.3687, -1.7647) -> (-18.583, -1.7518)
  line L515 (-18.583, -1.7518) -> (-18.7546, -1.7557)
  line L516 (-18.7546, -1.7557) -> (-18.9299, -1.7519)
  line L517 (-18.9299, -1.7519) -> (-19.2325, -1.7204)
  line L518 (-19.2325, -1.7204) -> (-19.4309, -1.6876)
  line L519 (-19.4309, -1.6876) -> (-19.6623, -1.6393)
  line L520 (-19.6623, -1.6393) -> (-19.9216, -1.5738)
  line L521 (-19.9216, -1.5738) -> (-20.2103, -1.4879)
  line L522 (-20.2103, -1.4879) -> (-20.5261, -1.3793)
  line L523 (-20.5261, -1.3793) -> (-20.8666, -1.2461)
  line L524 (-20.8666, -1.2461) -> (-21.2331, -1.0847)
  line L525 (-21.2331, -1.0847) -> (-21.6209, -0.8942)
  line L526 (-21.6209, -0.8942) -> (-21.989, -0.6945)
  arc A12 (-21.989, 0.6945) -> (-21.989, -0.6945) centre (0, 0) ccw
  line L527 (-21.989, 0.6945) -> (-21.6209, 0.8942)
  line L528 (-21.6209, 0.8942) -> (-21.2331, 1.0847)
  line L529 (-21.2331, 1.0847) -> (-20.8666, 1.2461)
  line L530 (-20.8666, 1.2461) -> (-20.5261, 1.3793)
  line L531 (-20.5261, 1.3793) -> (-20.2103, 1.4879)
  line L532 (-20.2103, 1.4879) -> (-19.9216, 1.5738)
  line L533 (-19.9216, 1.5738) -> (-19.6623, 1.6393)
  line L534 (-19.6623, 1.6393) -> (-19.4309, 1.6876)
  line L535 (-19.4309, 1.6876) -> (-19.2325, 1.7204)
  line L536 (-19.2325, 1.7204) -> (-18.9299, 1.7519)
  line L537 (-18.9299, 1.7519) -> (-18.7546, 1.7557)
  line L538 (-18.7546, 1.7557) -> (-18.583, 1.7518)
  line L539 (-18.583, 1.7518) -> (-18.3687, 1.7647)
  line L540 (-18.3687, 1.7647) -> (-18.1886, 1.7972)
  line L541 (-18.1886, 1.7972) -> (-18.1117, 1.8199)
  line L542 (-18.1117, 1.8199) -> (-18.0438, 1.8465)
  line L543 (-18.0438, 1.8465) -> (-17.985, 1.8765)
  line L544 (-17.985, 1.8765) -> (-17.9354, 1.9096)
  line L545 (-17.9354, 1.9096) -> (-17.8951, 1.9454)
  line L546 (-17.8951, 1.9454) -> (-17.8643, 1.9836)
  line L547 (-17.8643, 1.9836) -> (-17.8429, 2.0238)
  line L548 (-17.8429, 2.0238) -> (-17.8295, 2.0761)
  line L549 (-17.8295, 2.0761) -> (-17.7902, 2.3902)
  line L550 (-17.7902, 2.3902) -> (-17.729, 2.808)
  line L551 (-17.729, 2.808) -> (-17.6581, 3.2242)
  line L552 (-17.6581, 3.2242) -> (-17.5985, 3.5351)
  line L553 (-17.5985, 3.5351) -> (-17.5949, 3.589)
  line L554 (-17.5949, 3.589) -> (-17.6029, 3.6338)
  line L555 (-17.6029, 3.6338) -> (-17.6205, 3.6797)
  line L556 (-17.6205, 3.6797) -> (-17.6477, 3.7262)
  line L557 (-17.6477, 3.7262) -> (-17.6846, 3.773)
  line L558 (-17.6846, 3.773) -> (-17.7313, 3.8197)
  line L559 (-17.7313, 3.8197) -> (-17.7876, 3.866)
  line L560 (-17.7876, 3.866) -> (-17.8537, 3.9113)
  line L561 (-17.8537, 3.9113) -> (-18.015, 3.9979)
  line L562 (-18.015, 3.9979) -> (-18.2149, 4.0764)
  line L563 (-18.2149, 4.0764) -> (-18.3792, 4.1257)
  line L564 (-18.3792, 4.1257) -> (-18.5448, 4.1835)
  line L565 (-18.5448, 4.1835) -> (-18.8229, 4.307)
  line L566 (-18.8229, 4.307) -> (-19.0014, 4.3995)
  line L567 (-19.0014, 4.3995) -> (-19.2065, 4.5169)
  line L568 (-19.2065, 4.5169) -> (-19.4329, 4.6593)
  line L569 (-19.4329, 4.6593) -> (-19.6809, 4.8302)
  line L570 (-19.6809, 4.8302) -> (-19.9477, 5.0311)
  line L571 (-19.9477, 5.0311) -> (-20.2304, 5.263)
  line L572 (-20.2304, 5.263) -> (-20.5291, 5.5298)
  line L573 (-20.5291, 5.5298) -> (-20.839, 5.8308)
  line L574 (-20.839, 5.8308) -> (-21.1274, 6.1345)
  arc A13 (-20.6982, 7.4555) -> (-21.1274, 6.1345) centre (0, 0) ccw
  line L575 (-20.6982, 7.4555) -> (-20.2864, 7.5317)
  line L576 (-20.2864, 7.5317) -> (-19.8587, 7.593)
  line L577 (-19.8587, 7.593) -> (-19.4602, 7.6332)
  line L578 (-19.4602, 7.6332) -> (-19.0953, 7.6547)
  line L579 (-19.0953, 7.6547) -> (-18.7613, 7.6604)
  line L580 (-18.7613, 7.6604) -> (-18.4602, 7.6529)
  line L581 (-18.4602, 7.6529) -> (-18.1934, 7.6351)
  line L582 (-18.1934, 7.6351) -> (-17.9584, 7.6095)
  line L583 (-17.9584, 7.6095) -> (-17.7596, 7.5794)
  line L584 (-17.7596, 7.5794) -> (-17.462, 7.5158)
  line L585 (-17.462, 7.5158) -> (-17.2942, 7.4653)
  line L586 (-17.2942, 7.4653) -> (-17.1322, 7.4085)
  line L587 (-17.1322, 7.4085) -> (-16.9244, 7.3546)
  line L588 (-16.9244, 7.3546) -> (-16.743, 7.3298)
  line L589 (-16.743, 7.3298) -> (-16.6629, 7.3277)
  line L590 (-16.6629, 7.3277) -> (-16.5901, 7.3319)
  line L591 (-16.5901, 7.3319) -> (-16.5249, 7.3423)
  line L592 (-16.5249, 7.3423) -> (-16.4675, 7.3585)
  line L593 (-16.4675, 7.3585) -> (-16.4181, 7.3801)
  line L594 (-16.4181, 7.3801) -> (-16.3769, 7.4069)
  line L595 (-16.3769, 7.4069) -> (-16.3442, 7.4385)
  line L596 (-16.3442, 7.4385) -> (-16.3153, 7.4841)
  line L597 (-16.3153, 7.4841) -> (-16.1809, 7.7707)
  line L598 (-16.1809, 7.7707) -> (-15.9936, 8.1491)
  line L599 (-15.9936, 8.1491) -> (-15.7975, 8.5231)
  line L600 (-15.7975, 8.5231) -> (-15.6447, 8.8003)
  line L601 (-15.6447, 8.8003) -> (-15.6247, 8.8505)
  line L602 (-15.6247, 8.8505) -> (-15.6184, 8.8956)
  line L603 (-15.6184, 8.8956) -> (-15.621, 8.9446)
  line L604 (-15.621, 8.9446) -> (-15.6325, 8.9973)
  line L605 (-15.6325, 8.9973) -> (-15.6531, 9.0532)
  line L606 (-15.6531, 9.0532) -> (-15.6831, 9.112)
  line L607 (-15.6831, 9.112) -> (-15.7224, 9.1734)
  line L608 (-15.7224, 9.1734) -> (-15.7712, 9.237)
  line L609 (-15.7712, 9.237) -> (-15.8979, 9.3692)
  line L610 (-15.8979, 9.3692) -> (-16.0637, 9.5056)
  line L611 (-16.0637, 9.5056) -> (-16.2048, 9.6033)
  line L612 (-16.2048, 9.6033) -> (-16.3443, 9.7094)
  line L613 (-16.3443, 9.7094) -> (-16.5707, 9.9128)
  line L614 (-16.5707, 9.9128) -> (-16.7119, 10.0559)
  line L615 (-16.7119, 10.0559) -> (-16.8707, 10.231)
  line L616 (-16.8707, 10.231) -> (-17.042, 10.4364)
  line L617 (-17.042, 10.4364) -> (-17.225, 10.6756)
  line L618 (-17.225, 10.6756) -> (-17.4167, 10.9491)
  line L619 (-17.4167, 10.9491) -> (-17.6139, 11.257)
  line L620 (-17.6139, 11.257) -> (-17.8155, 11.603)
  line L621 (-17.8155, 11.603) -> (-18.0173, 11.985)
  line L622 (-18.0173, 11.985) -> (-18.1977, 12.3629)
  arc A14 (-17.3813, 13.4867) -> (-18.1977, 12.3629) centre (0, 0) ccw
  line L623 (-17.3813, 13.4867) -> (-16.9661, 13.4319)
  line L624 (-16.9661, 13.4319) -> (-16.5404, 13.3581)
  line L625 (-16.5404, 13.3581) -> (-16.149, 13.2732)
  line L626 (-16.149, 13.2732) -> (-15.7953, 13.1808)
  line L627 (-15.7953, 13.1808) -> (-15.4759, 13.083)
  line L628 (-15.4759, 13.083) -> (-15.1918, 12.9829)
  line L629 (-15.1918, 12.9829) -> (-14.9436, 12.8835)
  line L630 (-14.9436, 12.8835) -> (-14.728, 12.7865)
  line L631 (-14.728, 12.7865) -> (-14.5482, 12.6964)
  line L632 (-14.5482, 12.6964) -> (-14.2849, 12.544)
  line L633 (-14.2849, 12.544) -> (-14.1408, 12.4441)
  line L634 (-14.1408, 12.4441) -> (-14.0043, 12.3401)
  line L635 (-14.0043, 12.3401) -> (-13.8234, 12.2245)
  line L636 (-13.8234, 12.2245) -> (-13.6585, 12.1449)
  line L637 (-13.6585, 12.1449) -> (-13.5829, 12.1181)
  line L638 (-13.5829, 12.1181) -> (-13.5124, 12.0997)
  line L639 (-13.5124, 12.0997) -> (-13.4472, 12.0894)
  line L640 (-13.4472, 12.0894) -> (-13.3876, 12.0871)
  line L641 (-13.3876, 12.0871) -> (-13.334, 12.0924)
  line L642 (-13.334, 12.0924) -> (-13.2865, 12.1051)
  line L643 (-13.2865, 12.1051) -> (-13.2456, 12.125)
  line L644 (-13.2456, 12.125) -> (-13.2041, 12.1596)
  line L645 (-13.2041, 12.1596) -> (-12.9876, 12.3906)
  line L646 (-12.9876, 12.3906) -> (-12.6926, 12.6926)
  line L647 (-12.6926, 12.6926) -> (-12.3906, 12.9876)
  line L648 (-12.3906, 12.9876) -> (-12.1596, 13.2041)
  line L649 (-12.1596, 13.2041) -> (-12.125, 13.2456)
  line L650 (-12.125, 13.2456) -> (-12.1051, 13.2865)
  line L651 (-12.1051, 13.2865) -> (-12.0924, 13.334)
  line L652 (-12.0924, 13.334) -> (-12.0871, 13.3876)
  line L653 (-12.0871, 13.3876) -> (-12.0894, 13.4472)
  line L654 (-12.0894, 13.4472) -> (-12.0997, 13.5124)
  line L655 (-12.0997, 13.5124) -> (-12.1181, 13.5829)
  line L656 (-12.1181, 13.5829) -> (-12.1449, 13.6585)
  line L657 (-12.1449, 13.6585) -> (-12.2245, 13.8234)
  line L658 (-12.2245, 13.8234) -> (-12.3401, 14.0043)
  line L659 (-12.3401, 14.0043) -> (-12.4441, 14.1408)
  line L660 (-12.4441, 14.1408) -> (-12.544, 14.2849)
  line L661 (-12.544, 14.2849) -> (-12.6964, 14.5482)
  line L662 (-12.6964, 14.5482) -> (-12.7865, 14.728)
  line L663 (-12.7865, 14.728) -> (-12.8835, 14.9436)
  line L664 (-12.8835, 14.9436) -> (-12.9829, 15.1918)
  line L665 (-12.9829, 15.1918) -> (-13.083, 15.4759)
  line L666 (-13.083, 15.4759) -> (-13.1808, 15.7953)
  line L667 (-13.1808, 15.7953) -> (-13.2732, 16.149)
  line L668 (-13.2732, 16.149) -> (-13.3581, 16.5404)
  line L669 (-13.3581, 16.5404) -> (-13.4319, 16.9661)
  line L670 (-13.4319, 16.9661) -> (-13.4867, 17.3813)
  arc A15 (-12.3629, 18.1977) -> (-13.4867, 17.3813) centre (0, 0) ccw
  line L671 (-12.3629, 18.1977) -> (-11.985, 18.0173)
  line L672 (-11.985, 18.0173) -> (-11.603, 17.8155)
  line L673 (-11.603, 17.8155) -> (-11.257, 17.6139)
  line L674 (-11.257, 17.6139) -> (-10.9491, 17.4167)
  line L675 (-10.9491, 17.4167) -> (-10.6756, 17.225)
  line L676 (-10.6756, 17.225) -> (-10.4364, 17.042)
  line L677 (-10.4364, 17.042) -> (-10.231, 16.8707)
  line L678 (-10.231, 16.8707) -> (-10.0559, 16.7119)
  line L679 (-10.0559, 16.7119) -> (-9.9128, 16.5707)
  line L680 (-9.9128, 16.5707) -> (-9.7094, 16.3443)
  line L681 (-9.7094, 16.3443) -> (-9.6033, 16.2048)
  line L682 (-9.6033, 16.2048) -> (-9.5056, 16.0637)
  line L683 (-9.5056, 16.0637) -> (-9.3692, 15.8979)
  line L684 (-9.3692, 15.8979) -> (-9.237, 15.7712)
  line L685 (-9.237, 15.7712) -> (-9.1734, 15.7224)
  line L686 (-9.1734, 15.7224) -> (-9.112, 15.6831)
  line L687 (-9.112, 15.6831) -> (-9.0532, 15.6531)
  line L688 (-9.0532, 15.6531) -> (-8.9973, 15.6325)
  line L689 (-8.9973, 15.6325) -> (-8.9446, 15.621)
  line L690 (-8.9446, 15.621) -> (-8.8956, 15.6184)
  line L691 (-8.8956, 15.6184) -> (-8.8505, 15.6247)
  line L692 (-8.8505, 15.6247) -> (-8.8003, 15.6447)
  line L693 (-8.8003, 15.6447) -> (-8.5231, 15.7975)
  line L694 (-8.5231, 15.7975) -> (-8.1491, 15.9936)
  line L695 (-8.1491, 15.9936) -> (-7.7707, 16.1809)
  line L696 (-7.7707, 16.1809) -> (-7.4841, 16.3153)
  line L697 (-7.4841, 16.3153) -> (-7.4385, 16.3442)
  line L698 (-7.4385, 16.3442) -> (-7.4069, 16.3769)
  line L699 (-7.4069, 16.3769) -> (-7.3801, 16.4181)
  line L700 (-7.3801, 16.4181) -> (-7.3585, 16.4675)
  line L701 (-7.3585, 16.4675) -> (-7.3423, 16.5249)
  line L702 (-7.3423, 16.5249) -> (-7.3319, 16.5901)
  line L703 (-7.3319, 16.5901) -> (-7.3277, 16.6629)
  line L704 (-7.3277, 16.6629) -> (-7.3298, 16.743)
  line L705 (-7.3298, 16.743) -> (-7.3546, 16.9244)
  line L706 (-7.3546, 16.9244) -> (-7.4085, 17.1322)
  line L707 (-7.4085, 17.1322) -> (-7.4653, 17.2942)
  line L708 (-7.4653, 17.2942) -> (-7.5158, 17.462)
  line L709 (-7.5158, 17.462) -> (-7.5794, 17.7596)
  line L710 (-7.5794, 17.7596) -> (-7.6095, 17.9584)
  line L711 (-7.6095, 17.9584) -> (-7.6351, 18.1934)
  line L712 (-7.6351, 18.1934) -> (-7.6529, 18.4602)
  line L713 (-7.6529, 18.4602) -> (-7.6604, 18.7613)
  line L714 (-7.6604, 18.7613) -> (-7.6547, 19.0953)
  line L715 (-7.6547, 19.0953) -> (-7.6332, 19.4602)
  line L716 (-7.6332, 19.4602) -> (-7.593, 19.8587)
  line L717 (-7.593, 19.8587) -> (-7.5317, 20.2864)
  line L718 (-7.5317, 20.2864) -> (-7.4555, 20.6982)
  arc A16 (-6.1345, 21.1274) -> (-7.4555, 20.6982) centre (0, 0) ccw
  line L719 (-6.1345, 21.1274) -> (-5.8308, 20.839)
  line L720 (-5.8308, 20.839) -> (-5.5298, 20.5291)
  line L721 (-5.5298, 20.5291) -> (-5.263, 20.2304)
  line L722 (-5.263, 20.2304) -> (-5.0311, 19.9477)
  line L723 (-5.0311, 19.9477) -> (-4.8302, 19.6809)
  line L724 (-4.8302, 19.6809) -> (-4.6593, 19.4329)
  line L725 (-4.6593, 19.4329) -> (-4.5169, 19.2065)
  line L726 (-4.5169, 19.2065) -> (-4.3995, 19.0014)
  line L727 (-4.3995, 19.0014) -> (-4.307, 18.8229)
  line L728 (-4.307, 18.8229) -> (-4.1835, 18.5448)
  line L729 (-4.1835, 18.5448) -> (-4.1257, 18.3792)
  line L730 (-4.1257, 18.3792) -> (-4.0764, 18.2149)
  line L731 (-4.0764, 18.2149) -> (-3.9979, 18.015)
  line L732 (-3.9979, 18.015) -> (-3.9113, 17.8537)
  line L733 (-3.9113, 17.8537) -> (-3.866, 17.7876)
  line L734 (-3.866, 17.7876) -> (-3.8197, 17.7313)
  line L735 (-3.8197, 17.7313) -> (-3.773, 17.6846)
  line L736 (-3.773, 17.6846) -> (-3.7262, 17.6477)
  line L737 (-3.7262, 17.6477) -> (-3.6797, 17.6205)
  line L738 (-3.6797, 17.6205) -> (-3.6338, 17.6029)
  line L739 (-3.6338, 17.6029) -> (-3.589, 17.5949)
  line L740 (-3.589, 17.5949) -> (-3.5351, 17.5985)
  line L741 (-3.5351, 17.5985) -> (-3.2242, 17.6581)
  line L742 (-3.2242, 17.6581) -> (-2.808, 17.729)
  line L743 (-2.808, 17.729) -> (-2.3902, 17.7902)
  line L744 (-2.3902, 17.7902) -> (-2.0761, 17.8295)
  line L745 (-2.0761, 17.8295) -> (-2.0238, 17.8429)
  line L746 (-2.0238, 17.8429) -> (-1.9836, 17.8643)
  line L747 (-1.9836, 17.8643) -> (-1.9454, 17.8951)
  line L748 (-1.9454, 17.8951) -> (-1.9096, 17.9354)
  line L749 (-1.9096, 17.9354) -> (-1.8765, 17.985)
  line L750 (-1.8765, 17.985) -> (-1.8465, 18.0438)
  line L751 (-1.8465, 18.0438) -> (-1.8199, 18.1117)
  line L752 (-1.8199, 18.1117) -> (-1.7972, 18.1886)
  line L753 (-1.7972, 18.1886) -> (-1.7647, 18.3687)
  line L754 (-1.7647, 18.3687) -> (-1.7518, 18.583)
  line L755 (-1.7518, 18.583) -> (-1.7557, 18.7546)
  line L756 (-1.7557, 18.7546) -> (-1.7519, 18.9299)
  line L757 (-1.7519, 18.9299) -> (-1.7204, 19.2325)
  line L758 (-1.7204, 19.2325) -> (-1.6876, 19.4309)
  line L759 (-1.6876, 19.4309) -> (-1.6393, 19.6623)
  line L760 (-1.6393, 19.6623) -> (-1.5738, 19.9216)
  line L761 (-1.5738, 19.9216) -> (-1.4879, 20.2103)
  line L762 (-1.4879, 20.2103) -> (-1.3793, 20.5261)
  line L763 (-1.3793, 20.5261) -> (-1.2461, 20.8666)
  line L764 (-1.2461, 20.8666) -> (-1.0847, 21.2331)
  line L765 (-1.0847, 21.2331) -> (-0.8942, 21.6209)
  line L766 (-0.8942, 21.6209) -> (-0.6945, 21.989)
  arc A17 (0.6945, 21.989) -> (-0.6945, 21.989) centre (0, 0) ccw
  line L767 (0.6945, 21.989) -> (0.8942, 21.6209)
  line L768 (0.8942, 21.6209) -> (1.0847, 21.2331)
  line L769 (1.0847, 21.2331) -> (1.2461, 20.8666)
  line L770 (1.2461, 20.8666) -> (1.3793, 20.5261)
  line L771 (1.3793, 20.5261) -> (1.4879, 20.2103)
  line L772 (1.4879, 20.2103) -> (1.5738, 19.9216)
  line L773 (1.5738, 19.9216) -> (1.6393, 19.6623)
  line L774 (1.6393, 19.6623) -> (1.6876, 19.4309)
  line L775 (1.6876, 19.4309) -> (1.7204, 19.2325)
  line L776 (1.7204, 19.2325) -> (1.7519, 18.9299)
  line L777 (1.7519, 18.9299) -> (1.7557, 18.7546)
  line L778 (1.7557, 18.7546) -> (1.7518, 18.583)
  line L779 (1.7518, 18.583) -> (1.7647, 18.3687)
  line L780 (1.7647, 18.3687) -> (1.7972, 18.1886)
  line L781 (1.7972, 18.1886) -> (1.8199, 18.1117)
  line L782 (1.8199, 18.1117) -> (1.8465, 18.0438)
  line L783 (1.8465, 18.0438) -> (1.8765, 17.985)
  line L784 (1.8765, 17.985) -> (1.9096, 17.9354)
  line L785 (1.9096, 17.9354) -> (1.9454, 17.8951)
  line L786 (1.9454, 17.8951) -> (1.9836, 17.8643)
  line L787 (1.9836, 17.8643) -> (2.0238, 17.8429)
  line L788 (2.0238, 17.8429) -> (2.0761, 17.8295)
  line L789 (2.0761, 17.8295) -> (2.3902, 17.7902)
  line L790 (2.3902, 17.7902) -> (2.808, 17.729)
  line L791 (2.808, 17.729) -> (3.2242, 17.6581)
  line L792 (3.2242, 17.6581) -> (3.5351, 17.5985)
  line L793 (3.5351, 17.5985) -> (3.589, 17.5949)
  line L794 (3.589, 17.5949) -> (3.6338, 17.6029)
  line L795 (3.6338, 17.6029) -> (3.6797, 17.6205)
  line L796 (3.6797, 17.6205) -> (3.7262, 17.6477)
  line L797 (3.7262, 17.6477) -> (3.773, 17.6846)
  line L798 (3.773, 17.6846) -> (3.8197, 17.7313)
  line L799 (3.8197, 17.7313) -> (3.866, 17.7876)
  line L800 (3.866, 17.7876) -> (3.9113, 17.8537)
  line L801 (3.9113, 17.8537) -> (3.9979, 18.015)
  line L802 (3.9979, 18.015) -> (4.0764, 18.2149)
  line L803 (4.0764, 18.2149) -> (4.1257, 18.3792)
  line L804 (4.1257, 18.3792) -> (4.1835, 18.5448)
  line L805 (4.1835, 18.5448) -> (4.307, 18.8229)
  line L806 (4.307, 18.8229) -> (4.3995, 19.0014)
  line L807 (4.3995, 19.0014) -> (4.5169, 19.2065)
  line L808 (4.5169, 19.2065) -> (4.6593, 19.4329)
  line L809 (4.6593, 19.4329) -> (4.8302, 19.6809)
  line L810 (4.8302, 19.6809) -> (5.0311, 19.9477)
  line L811 (5.0311, 19.9477) -> (5.263, 20.2304)
  line L812 (5.263, 20.2304) -> (5.5298, 20.5291)
  line L813 (5.5298, 20.5291) -> (5.8308, 20.839)
  line L814 (5.8308, 20.839) -> (6.1345, 21.1274)
  arc A18 (7.4555, 20.6982) -> (6.1345, 21.1274) centre (0, 0) ccw
  line L815 (7.4555, 20.6982) -> (7.5317, 20.2864)
  line L816 (7.5317, 20.2864) -> (7.593, 19.8587)
  line L817 (7.593, 19.8587) -> (7.6332, 19.4602)
  line L818 (7.6332, 19.4602) -> (7.6547, 19.0953)
  line L819 (7.6547, 19.0953) -> (7.6604, 18.7613)
  line L820 (7.6604, 18.7613) -> (7.6529, 18.4602)
  line L821 (7.6529, 18.4602) -> (7.6351, 18.1934)
  line L822 (7.6351, 18.1934) -> (7.6095, 17.9584)
  line L823 (7.6095, 17.9584) -> (7.5794, 17.7596)
  line L824 (7.5794, 17.7596) -> (7.5158, 17.462)
  line L825 (7.5158, 17.462) -> (7.4653, 17.2942)
  line L826 (7.4653, 17.2942) -> (7.4085, 17.1322)
  line L827 (7.4085, 17.1322) -> (7.3546, 16.9244)
  line L828 (7.3546, 16.9244) -> (7.3298, 16.743)
  line L829 (7.3298, 16.743) -> (7.3277, 16.6629)
  line L830 (7.3277, 16.6629) -> (7.3319, 16.5901)
  line L831 (7.3319, 16.5901) -> (7.3423, 16.5249)
  line L832 (7.3423, 16.5249) -> (7.3585, 16.4675)
  line L833 (7.3585, 16.4675) -> (7.3801, 16.4181)
  line L834 (7.3801, 16.4181) -> (7.4069, 16.3769)
  line L835 (7.4069, 16.3769) -> (7.4385, 16.3442)
  line L836 (7.4385, 16.3442) -> (7.4841, 16.3153)
  line L837 (7.4841, 16.3153) -> (7.7707, 16.1809)
  line L838 (7.7707, 16.1809) -> (8.1491, 15.9936)
  line L839 (8.1491, 15.9936) -> (8.5231, 15.7975)
  line L840 (8.5231, 15.7975) -> (8.8003, 15.6447)
  line L841 (8.8003, 15.6447) -> (8.8505, 15.6247)
  line L842 (8.8505, 15.6247) -> (8.8956, 15.6184)
  line L843 (8.8956, 15.6184) -> (8.9446, 15.621)
  line L844 (8.9446, 15.621) -> (8.9973, 15.6325)
  line L845 (8.9973, 15.6325) -> (9.0532, 15.6531)
  line L846 (9.0532, 15.6531) -> (9.112, 15.6831)
  line L847 (9.112, 15.6831) -> (9.1734, 15.7224)
  line L848 (9.1734, 15.7224) -> (9.237, 15.7712)
  line L849 (9.237, 15.7712) -> (9.3692, 15.8979)
  line L850 (9.3692, 15.8979) -> (9.5056, 16.0637)
  line L851 (9.5056, 16.0637) -> (9.6033, 16.2048)
  line L852 (9.6033, 16.2048) -> (9.7094, 16.3443)
  line L853 (9.7094, 16.3443) -> (9.9128, 16.5707)
  line L854 (9.9128, 16.5707) -> (10.0559, 16.7119)
  line L855 (10.0559, 16.7119) -> (10.231, 16.8707)
  line L856 (10.231, 16.8707) -> (10.4364, 17.042)
  line L857 (10.4364, 17.042) -> (10.6756, 17.225)
  line L858 (10.6756, 17.225) -> (10.9491, 17.4167)
  line L859 (10.9491, 17.4167) -> (11.257, 17.6139)
  line L860 (11.257, 17.6139) -> (11.603, 17.8155)
  line L861 (11.603, 17.8155) -> (11.985, 18.0173)
  line L862 (11.985, 18.0173) -> (12.3629, 18.1977)
  arc A19 (13.4867, 17.3813) -> (12.3629, 18.1977) centre (0, 0) ccw
  line L863 (13.4867, 17.3813) -> (13.4319, 16.9661)
  line L864 (13.4319, 16.9661) -> (13.3581, 16.5404)
  line L865 (13.3581, 16.5404) -> (13.2732, 16.149)
  line L866 (13.2732, 16.149) -> (13.1808, 15.7953)
  line L867 (13.1808, 15.7953) -> (13.083, 15.4759)
  line L868 (13.083, 15.4759) -> (12.9829, 15.1918)
  line L869 (12.9829, 15.1918) -> (12.8835, 14.9436)
  line L870 (12.8835, 14.9436) -> (12.7865, 14.728)
  line L871 (12.7865, 14.728) -> (12.6964, 14.5482)
  line L872 (12.6964, 14.5482) -> (12.544, 14.2849)
  line L873 (12.544, 14.2849) -> (12.4441, 14.1408)
  line L874 (12.4441, 14.1408) -> (12.3401, 14.0043)
  line L875 (12.3401, 14.0043) -> (12.2245, 13.8234)
  line L876 (12.2245, 13.8234) -> (12.1449, 13.6585)
  line L877 (12.1449, 13.6585) -> (12.1181, 13.5829)
  line L878 (12.1181, 13.5829) -> (12.0997, 13.5124)
  line L879 (12.0997, 13.5124) -> (12.0894, 13.4472)
  line L880 (12.0894, 13.4472) -> (12.0871, 13.3876)
  line L881 (12.0871, 13.3876) -> (12.0924, 13.334)
  line L882 (12.0924, 13.334) -> (12.1051, 13.2865)
  line L883 (12.1051, 13.2865) -> (12.125, 13.2456)
  line L884 (12.125, 13.2456) -> (12.1596, 13.2041)
  line L885 (12.1596, 13.2041) -> (12.3906, 12.9876)
  line L886 (12.3906, 12.9876) -> (12.6926, 12.6926)
  line L887 (12.6926, 12.6926) -> (12.9876, 12.3906)
  line L888 (12.9876, 12.3906) -> (13.2041, 12.1596)
  line L889 (13.2041, 12.1596) -> (13.2456, 12.125)
  line L890 (13.2456, 12.125) -> (13.2865, 12.1051)
  line L891 (13.2865, 12.1051) -> (13.334, 12.0924)
  line L892 (13.334, 12.0924) -> (13.3876, 12.0871)
  line L893 (13.3876, 12.0871) -> (13.4472, 12.0894)
  line L894 (13.4472, 12.0894) -> (13.5124, 12.0997)
  line L895 (13.5124, 12.0997) -> (13.5829, 12.1181)
  line L896 (13.5829, 12.1181) -> (13.6585, 12.1449)
  line L897 (13.6585, 12.1449) -> (13.8234, 12.2245)
  line L898 (13.8234, 12.2245) -> (14.0043, 12.3401)
  line L899 (14.0043, 12.3401) -> (14.1408, 12.4441)
  line L900 (14.1408, 12.4441) -> (14.2849, 12.544)
  line L901 (14.2849, 12.544) -> (14.5482, 12.6964)
  line L902 (14.5482, 12.6964) -> (14.728, 12.7865)
  line L903 (14.728, 12.7865) -> (14.9436, 12.8835)
  line L904 (14.9436, 12.8835) -> (15.1918, 12.9829)